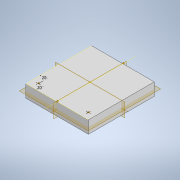
# Autodesk Inventor part: hub
Saved by Autodesk Inventor 2021 (Build 250183000, 183)
## iProperties
Created: 2021-05-06
Part Number: hub
Material: Generic
Document SubType Name: Modeling
Designer: andre
Density: 1 g/cm^3
Appearance: Default
Author: andre
Autodesk Inventor part; units mm, degrees
sketch "Sketch1" plane through (0, 0, 0) normal (0, 1, 0) x (-1, 0, 0)
  line L0 (-100, 105) -> (100, 105)
  line L1 (100, 105) -> (100, -105)
  line L2 (100, -105) -> (-100, -105)
  line L3 (-100, -105) -> (-100, 105)
  line L4 (-100, 105) -> (100, -105) construction
  line L5 (100, 105) -> (-100, -105) construction
  point P0 (0, 0)
  dimension "d0" = 200
  dimension "d1" = 210
  constraints: 12 end point, 2 midpoint, 2 parallel, 1 horizontal, 1 perpendicular
  measures "d0" distance of L1.end L2.end
  measures "d1" distance of L0.end L1.end
extrude "Extrusion1" add sketch "Sketch1" against normal mid plane 40
sketch "Sketch3" plane through (0, 20, 0) normal (0, 1, 0) x (1, 0, 0)
  line L0 (-100, 105) -> (-100, -105) construction
  line L1 (-100, -105) -> (100, -105) construction
  line L2 (0, 147) -> (0, -147) construction
  point P0 (0, 0)
  point P1 (-80, -85)
  point P2 (80, -85)
  dimension "d5" = 20
  dimension "d6" = 20
  constraints: 1 symmetric about line
  measures "d5" distance from line of L0 point (-80, -85)
  measures "d6" distance from line of point (-80, -85) L1
body "Solid1"
